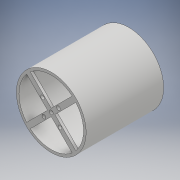
# Autodesk Inventor part: 零件2
Saved by Autodesk Inventor 2017 (Build 210142000, 142)
## iProperties
Part Number: 零件2
Material: 一般
Document SubType Name: Modeling
Designer: user
Density: 1 g/cm^3
Appearance: 預設
Author: user
Autodesk Inventor part; units mm, degrees
ref_plane "YZ Plane" through (0, 0, 0) normal (1, 0, 0) x (0, 1, 0)
ref_plane "XZ Plane" through (0, 0, 0) normal (0, 1, 0) x (-1, 0, 0)
ref_plane "XY Plane" through (0, 0, 0) normal (0, 0, 1) x (1, 0, 0)
sketch "草圖1" plane through (0, 0, 0) normal (0, 1, 0) x (-1, 0, 0)
  circle A0 centre (0, 0) radius 25
  circle A1 centre (0, 0) radius 27
  dimension "d0" = 50
  dimension "d1" = 2
  constraints: 2 centre point, 2 coincident
  measures "d0" diameter of A0
  measures "d1" radial gap between concentric circles of A0 A1
extrude "擠出1" add sketch "草圖1" along normal blind 60
sketch "草圖2" plane through (0, 0, 0) normal (0, -1, 0) x (1, 0, 0)
  circle A0 centre (0, 0) radius 25 construction
  line L0 (-25, 0) -> (25, 0) construction
  line L1 (-17.6777, 17.6777) -> (17.6777, -17.6777) construction
  line L2 (-16.2068, 19.0352) -> (19.0352, -16.2068)
  line L3 (-19.0352, 16.2068) -> (16.2068, -19.0352)
  arc A1 (-16.2068, 19.0352) -> (-19.0352, 16.2068) centre (0, 0) ccw
  arc A2 (16.2068, -19.0352) -> (19.0352, -16.2068) centre (0, 0) ccw
  line L4 (-19.0352, -16.2068) -> (16.2068, 19.0352)
  arc A3 (-19.0352, -16.2068) -> (-16.2068, -19.0352) centre (0, 0) ccw
  line L5 (-16.2068, -19.0352) -> (19.0352, 16.2068)
  arc A4 (19.0352, 16.2068) -> (16.2068, 19.0352) centre (0, 0) ccw
  dimension "d10" = 45
  dimension "d11" = 2
  dimension "d14" = 90
  constraints: 14 point on circle, 12 end point, 4 centre point, 2 midpoint, 2 symmetric about line, 1 coincident, 1 horizontal, 1 parallel, 10 other
  measures "d10" angle of L0 L1
  measures "d11" distance between parallel lines of L1 L2
extrude "擠出3" add sketch "草圖2" against normal blind 2
sketch "草圖5" plane through (0, 0, 0) normal (0, -1, 0) x (1, 0, 0)
  circle A0 centre (0, 0) radius 25 construction
  line L0 (17.6777, 17.6777) -> (-17.6777, -17.6777) construction
  line L1 (-17.6777, 17.6777) -> (17.6777, -17.6777) construction
  line L2 (-25, 0) -> (25, 0) construction
  arc A1 (19.0352, -16.2068) -> (19.0352, 16.2068) centre (0, 0) ccw construction
  point P0 (5.6569, 5.6569)
  point P1 (-6.7175, 6.7175)
  point P2 (0, 0)
  point P3 (-5.6569, -5.6569)
  point P4 (6.7175, -6.7175)
  dimension "d18" = 45
  dimension "d19" = 45
  dimension "d20" = 9.5
  dimension "d21" = 8
  dimension "d24" = 180
  constraints: 6 end point, 3 midpoint, 2 point on line, 1 coincident, 1 horizontal, 1 point on circle, 10 other
  measures "d18" angle of L2 L0
  measures "d19" angle of L2 L1
  measures "d20" distance from line of L0 point (-6.718, 6.718)
  measures "d21" distance from line of L1 point (5.657, 5.657)
hole "孔1" at (0, 0, 0) at (5.6569, 0, 5.6569) at (-6.7175, 0, 6.7175) at (-5.6569, 0, -5.6569) at (6.7175, 0, -6.7175) direction (0, 1, 0) diameter 3 end through all
